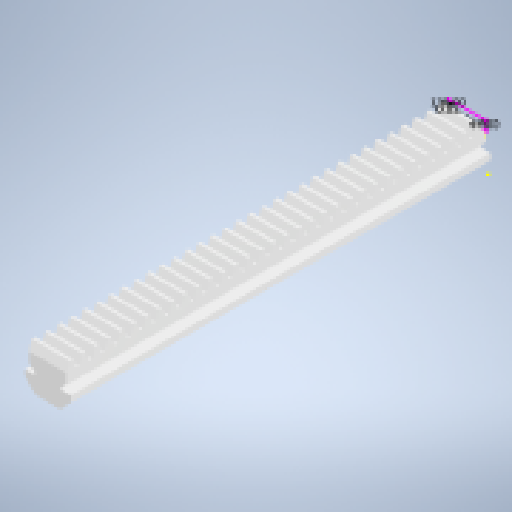
# Autodesk Inventor part: test_extrusion_rack
Saved by Autodesk Inventor 2023.2 (Build 272271000, 271)
## iProperties
Created: 2023-02-15
Part Number: test_extrusion_rack
Material: ABS Plastic
Document SubType Name: Modeling
Designer: dmargari
Density: 1.06 g/cm^3
Appearance: Smooth - White
Author: dmargari
## iProperties of the stored document test_extrusion_rack_3DPrint.ipt
Created: 2023-02-15
Part Number: test_extrusion_rack_3DPrint
Material: Generic
Document SubType Name: Modeling
Designer: dmargari
Density: 1 g/cm^3
Appearance: Default
Author: dmargari
Autodesk Inventor part; units mm, degrees
ref_plane "YZ Plane" through (0, 0, 0) normal (1, 0, 0) x (0, 1, 0)
ref_plane "XZ Plane" through (0, 0, 0) normal (0, 1, 0) x (-1, 0, 0)
ref_plane "XY Plane" through (0, 0, 0) normal (0, 0, 1) x (1, 0, 0)
sketch "Sketch1" plane through (0, 0, 0) normal (0, 0, 1) x (1, 0, 0)
  arc A0 (-8.2084, 4.5843) -> (-8.067, 4.9257) centre (-8.2084, 4.7843) ccw
  line L0 (-7.7495, 0.3197) -> (-10.4102, 2.9803)
  line L1 (-8.067, 4.9257) -> (-9.3477, 6.2065)
  line L2 (-10.4102, 2.9803) -> (-10.4102, 4.5843)
  line L3 (-10.4102, 4.5843) -> (-8.2084, 4.5843)
  line L4 (-5.115, 0.3197) -> (-7.7495, 0.3197)
  line L5 (-9.3477, 6.2065) -> (-0.5433, 6.2065)
  line L6 (-4.9102, 0.1149) -> (-5.115, 0.3197)
  line L7 (-4.7054, 0.3197) -> (-4.9102, 0.1149)
  line L8 (-2.0001, 0.3197) -> (-4.7054, 0.3197)
  arc A1 (-1.7888, 5.0111) -> (-1.6473, 4.6697) centre (-1.6473, 4.8697) ccw
  line L9 (-0.5433, 6.2065) -> (-1.7888, 5.0111)
  line L10 (-0.5433, 6.2065) -> (-1.7888, 5.0111)
  line L11 (-1.6473, 4.6697) -> (0.6398, 4.6697)
  line L12 (0.6398, 4.6697) -> (0.6398, 2.9596)
  line L13 (0.6398, 2.9596) -> (-2.0001, 0.3197)
  line L14 (-5.115, 0.3197) -> (-4.7054, 0.3197)
  line L15 (-9.3477, 6.2065) -> (-9.3477, 8.5065)
  line L16 (-0.5433, 8.3065) -> (-0.5433, 6.2065)
  arc A2 (-1.8948, 5.1172) -> (-1.6473, 4.5197) centre (-1.6473, 4.8697) ccw
  line L17 (-1.6473, 4.5197) -> (0.4898, 4.5197)
  line L18 (0.4898, 4.5197) -> (0.4898, 3.0217)
  line L19 (0.4898, 3.0217) -> (-2.0623, 0.4697)
  line L20 (-2.0623, 0.4697) -> (-4.9348, 0.4697)
  line L21 (-5.115, 0.4697) -> (-7.6874, 0.4697)
  line L22 (-7.6874, 0.4697) -> (-10.2602, 3.0425)
  line L23 (-10.2602, 3.0425) -> (-10.2602, 4.4343)
  line L24 (-10.2602, 4.4343) -> (-8.2084, 4.4343)
  arc A3 (-8.2084, 4.4343) -> (-7.9609, 5.0318) centre (-8.2084, 4.7843) ccw
  line L25 (-7.9609, 5.0318) -> (-9.2417, 6.3126)
  line L26 (-0.6472, 6.3147) -> (-1.8926, 5.1193)
  line L27 (-1.8926, 5.1193) -> (-1.8948, 5.1172)
  line L28 (-0.6472, 6.3147) -> (-0.5433, 6.3147)
  line L29 (-9.2417, 6.3126) -> (-9.3477, 6.3147)
  line L30 (-4.9348, 0.4697) -> (-5.115, 0.4697)
  line L31 (-0.5433, 8.3065) -> (-0.5433, 10.6065)
  line L32 (-0.5433, 10.6065) -> (-9.3477, 10.6065)
  line L33 (-9.3477, 10.6065) -> (-9.3477, 8.5065)
  point P0 (0, 0)
  point P1 (-9.3477, 6.3442)
  point P2 (-0.76, 6.2065)
  point P3 (-9.1356, 6.2065)
  dimension "d9" = 0.15
  dimension "d10" = 0.15
  dimension "d11" = 0.15
  dimension "d68" = 4.4
  constraints: 68 end point, 8 point on circle, 4 centre point, 4 perpendicular, 4 point on line, 2 collinear, 1 horizontal, 1 parallel, 1 vertical, 9 other
  measures "d9" radial gap between concentric circles of A1 A2
  measures "d10" distance between parallel lines of L4 L21
  measures "d11" distance between parallel lines of L9 L26
  measures "d68" distance between parallel lines of L32 L5
extrude "Extrusion3" add sketch "Sketch1" along normal blind 98.27 contours L15 L29 L25 L5 | L25 L29 L15 L33 L32 L31 L16 L28 L26 L5 | L5 L26 L27 A2 L17 L18 L19 L20 L30 L21 L22 L23 L24 A3 L25 | L26 L28 L16 L5
sketch "Sketch5" plane through (0, 0, 0) normal (0, 0, -1) x (-1, 0, 0)
  line L0 (9.3477, 8.5065) -> (0.5433, 8.5065) projected
  line L1 (9.3477, 8.5065) -> (9.3477, 10.6065) construction
  line L2 (9.3477, 9.3565) -> (0.2216, 9.3565) construction
  line L3 (9.3477, 9.3565) -> (11.1472, 9.3565) construction
  line L4 (0.2216, 9.3565) -> (2.0211, 9.3565) construction
  line L5 (0.5433, 6.2065) -> (0.5433, 10.6065) construction
  line L6 (0.5433, 9.3565) -> (2.3428, 9.3565) construction
  line L7 (0.5433, 10.6065) -> (9.3477, 10.6065) projected
  line L8 (0.5433, 9.3565) -> (1.8378, 10.6065)
  line L9 (0.5433, 10.6065) -> (9.3477, 10.6065) projected
  line L10 (0.5433, 9.3565) -> (2.3428, 9.3565) construction
  line L11 (9.3477, 9.3565) -> (8.0533, 10.6065)
  line L12 (9.3477, 9.3565) -> (11.1472, 9.3565) construction
  line L13 (9.3477, 10.6065) -> (9.3477, 8.5065) projected
  line L14 (9.3477, 10.6065) -> (9.3477, 9.3565)
  line L15 (0.5433, 10.6065) -> (0.5433, 8.5065) projected
  line L16 (0.5433, 9.3565) -> (0.5433, 10.6065)
  point P0 (0, 0)
  point P1 (0.5433, 9.8936)
  point P2 (8.0533, 10.6065)
  point P3 (1.8378, 10.6065)
  dimension "d32" = 0.85
  dimension "d36" = 44
  dimension "d37" = 136
  constraints: 20 end point, 6 horizontal, 5 point on line, 2 collinear, 2 equal length
  measures "d32" distance from line of L0.start L2
  measures "d36" angle of L10 L8
  measures "d37" angle of L12 L11
sketch "Sketch7" plane through (-9.3477, 6.2065, 0) normal (-1, 0, 0) x (0, 0, 1)
  line L0 (0, 4.4) -> (0, 0) construction
  line L1 (0, 2.3) -> (102.4, 2.3) construction
  line L2 (0, 0) -> (98.27, 0) construction
  line L3 (0, 2.3) -> (0.672, 2.3)
  line L4 (0.672, 2.3) -> (1.4363, 4.4)
  line L5 (0, 4.4) -> (98.27, 4.4) projected
  line L6 (0.672, 2.3) -> (2.9068, 2.3) construction
  line L7 (1.4363, 4.4) -> (2.214, 4.4)
  line L8 (2.214, 4.4) -> (2.9784, 2.3)
  line L9 (2.214, 4.4) -> (4.4488, 4.4) construction
  line L10 (2.978, 2.3) -> (3.65, 2.3)
  line L11 (3.65, 2.3) -> (4.4143, 4.4)
  line L12 (5.192, 4.4) -> (5.9564, 2.3)
  line L13 (5.956, 2.3) -> (6.628, 2.3)
  line L14 (6.628, 2.3) -> (7.3923, 4.4)
  line L15 (8.17, 4.4) -> (8.9344, 2.3)
  line L16 (8.934, 2.3) -> (9.606, 2.3)
  line L17 (9.606, 2.3) -> (10.3703, 4.4)
  line L18 (11.148, 4.4) -> (11.9124, 2.3)
  line L19 (11.912, 2.3) -> (12.584, 2.3)
  line L20 (12.584, 2.3) -> (13.3483, 4.4)
  line L21 (14.126, 4.4) -> (14.8904, 2.3)
  line L22 (14.89, 2.3) -> (15.562, 2.3)
  line L23 (15.562, 2.3) -> (16.3263, 4.4)
  line L24 (17.104, 4.4) -> (17.8684, 2.3)
  line L25 (17.868, 2.3) -> (18.54, 2.3)
  line L26 (18.54, 2.3) -> (19.3043, 4.4)
  line L27 (20.082, 4.4) -> (20.8464, 2.3)
  line L28 (20.846, 2.3) -> (21.518, 2.3)
  line L29 (21.518, 2.3) -> (22.2823, 4.4)
  line L30 (23.06, 4.4) -> (23.8244, 2.3)
  line L31 (23.824, 2.3) -> (24.496, 2.3)
  line L32 (24.496, 2.3) -> (25.2603, 4.4)
  line L33 (26.038, 4.4) -> (26.8024, 2.3)
  line L34 (26.802, 2.3) -> (27.474, 2.3)
  line L35 (27.474, 2.3) -> (28.2383, 4.4)
  line L36 (29.016, 4.4) -> (29.7804, 2.3)
  line L37 (29.78, 2.3) -> (30.452, 2.3)
  line L38 (30.452, 2.3) -> (31.2163, 4.4)
  line L39 (31.994, 4.4) -> (32.7584, 2.3)
  line L40 (32.758, 2.3) -> (33.43, 2.3)
  line L41 (33.43, 2.3) -> (34.1943, 4.4)
  line L42 (34.972, 4.4) -> (35.7364, 2.3)
  line L43 (35.736, 2.3) -> (36.408, 2.3)
  line L44 (36.408, 2.3) -> (37.1723, 4.4)
  line L45 (37.95, 4.4) -> (38.7144, 2.3)
  line L46 (38.714, 2.3) -> (39.386, 2.3)
  line L47 (39.386, 2.3) -> (40.1503, 4.4)
  line L48 (40.928, 4.4) -> (41.6924, 2.3)
  line L49 (41.692, 2.3) -> (42.364, 2.3)
  line L50 (42.364, 2.3) -> (43.1283, 4.4)
  line L51 (43.906, 4.4) -> (44.6704, 2.3)
  line L52 (44.67, 2.3) -> (45.342, 2.3)
  line L53 (45.342, 2.3) -> (46.1063, 4.4)
  line L54 (46.884, 4.4) -> (47.6484, 2.3)
  line L55 (47.648, 2.3) -> (48.32, 2.3)
  line L56 (48.32, 2.3) -> (49.0843, 4.4)
  line L57 (49.862, 4.4) -> (50.6264, 2.3)
  line L58 (50.626, 2.3) -> (51.298, 2.3)
  line L59 (51.298, 2.3) -> (52.0623, 4.4)
  line L60 (52.84, 4.4) -> (53.6044, 2.3)
  line L61 (53.604, 2.3) -> (54.276, 2.3)
  line L62 (54.276, 2.3) -> (55.0403, 4.4)
  line L63 (55.818, 4.4) -> (56.5824, 2.3)
  line L64 (56.582, 2.3) -> (57.254, 2.3)
  line L65 (57.254, 2.3) -> (58.0183, 4.4)
  line L66 (58.796, 4.4) -> (59.5604, 2.3)
  line L67 (59.56, 2.3) -> (60.232, 2.3)
  line L68 (60.232, 2.3) -> (60.9963, 4.4)
  line L69 (61.774, 4.4) -> (62.5384, 2.3)
  line L70 (62.538, 2.3) -> (63.21, 2.3)
  line L71 (63.21, 2.3) -> (63.9743, 4.4)
  line L72 (64.752, 4.4) -> (65.5164, 2.3)
  line L73 (65.516, 2.3) -> (66.188, 2.3)
  line L74 (66.188, 2.3) -> (66.9523, 4.4)
  line L75 (67.73, 4.4) -> (68.4944, 2.3)
  line L76 (68.494, 2.3) -> (69.166, 2.3)
  line L77 (69.166, 2.3) -> (69.9303, 4.4)
  line L78 (70.708, 4.4) -> (71.4724, 2.3)
  line L79 (71.472, 2.3) -> (72.144, 2.3)
  line L80 (72.144, 2.3) -> (72.9083, 4.4)
  line L81 (73.686, 4.4) -> (74.4504, 2.3)
  line L82 (74.45, 2.3) -> (75.122, 2.3)
  line L83 (75.122, 2.3) -> (75.8863, 4.4)
  line L84 (76.664, 4.4) -> (77.4284, 2.3)
  line L85 (77.428, 2.3) -> (78.1, 2.3)
  line L86 (78.1, 2.3) -> (78.8643, 4.4)
  line L87 (79.642, 4.4) -> (80.4064, 2.3)
  line L88 (80.406, 2.3) -> (81.078, 2.3)
  line L89 (81.078, 2.3) -> (81.8423, 4.4)
  line L90 (82.62, 4.4) -> (83.3844, 2.3)
  line L91 (83.384, 2.3) -> (84.056, 2.3)
  line L92 (84.056, 2.3) -> (84.8203, 4.4)
  line L93 (85.598, 4.4) -> (86.3624, 2.3)
  line L94 (86.362, 2.3) -> (87.034, 2.3)
  line L95 (87.034, 2.3) -> (87.7983, 4.4)
  line L96 (88.576, 4.4) -> (89.3404, 2.3)
  line L97 (89.34, 2.3) -> (90.012, 2.3)
  line L98 (90.012, 2.3) -> (90.7763, 4.4)
  line L99 (91.554, 4.4) -> (92.3184, 2.3)
  line L100 (92.318, 2.3) -> (92.99, 2.3)
  line L101 (92.99, 2.3) -> (93.7543, 4.4)
  line L102 (94.532, 4.4) -> (95.2964, 2.3)
  line L103 (95.296, 2.3) -> (95.968, 2.3)
  line L104 (95.968, 2.3) -> (96.7323, 4.4)
  line L105 (97.51, 4.4) -> (98.2744, 2.3)
  line L106 (0, 4.4) -> (0, 0) projected
  line L107 (0, 0) -> (98.27, 0) projected
  line L108 (98.27, 4.4) -> (98.27, 0) projected
  line L109 (0, 4.4) -> (98.27, 4.4) projected
  point P0 (0, -6.2065)
  point P1 (0, 3.15)
  point P2 (98.27, 2.312)
  point P3 (95.2964, 2.3)
  point P4 (92.3184, 2.3)
  point P5 (89.3404, 2.3)
  point P6 (86.3624, 2.3)
  point P7 (80.4064, 2.3)
  point P8 (83.3844, 2.3)
  point P9 (77.4284, 2.3)
  point P10 (74.4504, 2.3)
  point P11 (65.5164, 2.3)
  point P12 (71.4724, 2.3)
  point P13 (68.4944, 2.3)
  point P14 (62.5384, 2.3)
  point P15 (59.5604, 2.3)
  point P16 (56.5824, 2.3)
  point P17 (53.6044, 2.3)
  point P18 (50.6264, 2.3)
  point P19 (47.6484, 2.3)
  point P20 (44.6704, 2.3)
  point P21 (41.6924, 2.3)
  point P22 (38.7144, 2.3)
  point P23 (35.7364, 2.3)
  point P24 (32.7584, 2.3)
  point P25 (29.7804, 2.3)
  point P26 (26.8024, 2.3)
  point P27 (23.8244, 2.3)
  point P28 (20.8464, 2.3)
  point P29 (17.8684, 2.3)
  point P30 (14.8904, 2.3)
  point P31 (11.9124, 2.3)
  point P32 (8.9344, 2.3)
  point P33 (5.9564, 2.3)
  point P34 (2.9784, 2.3)
  dimension "d69" = 2.3
  dimension "d70" = 0.672
  dimension "d71" = 70
  dimension "d72" = 70
  dimension "d73" = 2.9784
  dimension "d76" = 2.978
  constraints: 206 end point, 4 horizontal, 3 point on line, 2 equal length, 259 other
  measures "d69" distance between parallel lines of L1 L2
  measures "d70" distance of L1.start L3.end
  measures "d71" angle of L6 L4
  measures "d72" angle of L8 L9
  measures "d73" distance of L8.end L1.start
  measures "d76" distance of L1.start L10.start
extrude "Extrusion7" cut sketch "Sketch7" against normal blind 98.27 contours L106 L5 L4 L3 | L5 L11 L10 L8 | L105 L5 L108 | L5 L14 L13 L12 | L104 L103 L102 L5 | L5 L17 L16 L15 | L101 L100 L99 L5 | L5 L20 L19 L18 | L98 L97 L96 L5 | L5 L23 L22 L21 | L95 L94 L93 L5 | L5 L26 L25 L24 | L92 L91 L90 L5 | L5 L29 L28 L27 | L89 L88 L87 L5 | L5 L32 L31 L30 | L86 L85 L84 L5 | L5 L35 L34 L33 | L83 L82 L81 L5 | L5 L38 L37 L36 | L80 L79 L78 L5 | L5 L41 L40 L39 | L77 L76 L75 L5 | L5 L44 L43 L42 | L74 L73 L72 L5 | L5 L47 L46 L45 | L71 L70 L69 L5 | L5 L50 L49 L48 | L68 L67 L66 L5 | L5 L53 L52 L51 | L65 L64 L63 L5 | L5 L56 L55 L54 | L62 L61 L60 L5 | L5 L59 L58 L57
body "Solid3"
